test in  siriys xy (Autodesk Fusion 360 design; units mm, degrees)
Autodesk Fusion 360 part; units mm, degrees
note: some values were not read from the file. Set by a fixed rule: which sketch regions a step uses.
(part 1 of 2)
sketch "sdfjkvcsd" plane through (0, 0, 0) normal (0, 0, 1) x (1, 0, 0)
  line L0 (-177.8, 0) -> (0, 0)
  line L1 (-177.7996, 0.7937) -> (-177.8, 0)
  line L2 (0, 1.5875) -> (0.0008, 16.3703)
  line L3 (0.0008, 16.3703) -> (0, 48.914)
  line L4 (0, 48.914) -> (0, 81.4578)
  line L5 (0.0008, 101.1047) -> (0, 161.4297)
  line L6 (-177.8, 177.8) -> (-177.8, 1.5875)
  line L7 (0, 161.4297) -> (0.0008, 166.6875)
  line L8 (-177.8, 1.5875) -> (-177.7996, 0.7937)
  line L9 (0, 81.4578) -> (0.0008, 101.1047)
  line L10 (0, 0) -> (0, 1.5875)
  line L11 (0.0008, 166.6875) -> (0, 177.8)
  line L12 (0, 177.8) -> (-177.8, 177.8)
  line L13 (-157.7594, 165.1) -> (-134.3406, 165.1)
  line L14 (-134.3406, 114.3) -> (-157.7594, 114.3)
  line L15 (-157.7594, 114.3) -> (-157.7594, 165.1)
  line L16 (-134.3406, 165.1) -> (-134.3406, 114.3)
  line L17 (-76.0757, 98.8543) -> (-75.9232, 99.2225)
  line L18 (-25.4, 77.1906) -> (-73.6593, 77.1906)
  line L19 (-74.8124, 77.4674) -> (-75.153, 77.6757)
  line L20 (-75.7149, 99.5624) -> (-75.4561, 99.8654)
  line L21 (-74.4449, 77.3149) -> (-74.8124, 77.4674)
  line L22 (-74.0573, 77.2219) -> (-74.4449, 77.3149)
  line L23 (-75.7149, 78.2376) -> (-75.9232, 78.5775)
  line L24 (-75.9232, 99.2225) -> (-75.7149, 99.5624)
  line L25 (-75.153, 100.1243) -> (-74.8131, 100.3326)
  line L26 (-76.2, 79.7306) -> (-76.2, 98.0694)
  line L27 (-74.4449, 100.4851) -> (-74.0573, 100.5781)
  line L28 (-76.1687, 79.3333) -> (-76.2, 79.7306)
  line L29 (-75.153, 77.6757) -> (-75.4561, 77.9345)
  line L30 (-76.168, 98.4667) -> (-76.0757, 98.8543)
  line L31 (-75.4561, 99.8654) -> (-75.153, 100.1243)
  line L32 (-75.4561, 77.9345) -> (-75.7149, 78.2376)
  line L33 (-25.4, 100.6094) -> (-25.4, 77.1906)
  line L34 (-76.0757, 78.9457) -> (-76.1687, 79.3333)
  line L35 (-73.6593, 77.1906) -> (-74.0573, 77.2219)
  line L36 (-73.6593, 100.6094) -> (-25.4, 100.6094)
  line L37 (-74.8131, 100.3326) -> (-74.4449, 100.4851)
  line L38 (-74.0573, 100.5781) -> (-73.6593, 100.6094)
  line L39 (-75.9232, 78.5775) -> (-76.0757, 78.9457)
  line L40 (-76.2, 98.0694) -> (-76.168, 98.4667)
  line L41 (-75.7149, 75.153) -> (-75.4561, 75.456)
  line L42 (-75.1484, 75.7193) -> (-74.8086, 75.9276)
  line L43 (-76.1687, 74.0573) -> (-76.0757, 74.4449)
  line L44 (-26.0553, 73.1777) -> (-26.393, 72.9362)
  line L45 (-76.2, 73.6592) -> (-76.1687, 74.0573)
  line L46 (-76.2, 19.0544) -> (-76.2, 73.6592)
  line L47 (-75.3736, 75.5265) -> (-75.1484, 75.7193)
  line L48 (-75.9232, 74.8131) -> (-75.7149, 75.153)
  line L49 (-165.0955, 19.0544) -> (-76.2, 19.0544)
  line L50 (-74.0528, 76.1732) -> (-73.6555, 76.2037)
  line L51 (-165.0955, 19.05) -> (-165.0955, 19.0544)
  line L52 (-73.6555, 76.2037) -> (-25.3955, 76.2037)
  line L53 (-74.8086, 75.9276) -> (-74.4404, 76.0801)
  line L54 (-25.1866, 75.4706) -> (-25.1734, 75.4034)
  line L55 (-25.3355, 74.1805) -> (-25.4586, 73.9313)
  line L56 (-25.7615, 73.471) -> (-26.0553, 73.1777)
  line L57 (-25.5194, 73.809) -> (-25.7615, 73.471)
  line L58 (-75.4561, 75.456) -> (-75.3736, 75.5265)
  line L59 (-25.2531, 75.8137) -> (-25.2252, 75.6655)
  line L60 (-25.1602, 74.9892) -> (-25.2147, 74.5776)
  line L61 (-74.4404, 76.0801) -> (-74.0528, 76.1732)
  line L62 (-25.2147, 74.5776) -> (-25.3355, 74.1805)
  line L63 (-25.1734, 75.4034) -> (-25.1602, 74.9892)
  line L64 (-25.4586, 73.9313) -> (-25.5194, 73.809)
  line L65 (-25.3955, 76.2037) -> (-25.2531, 75.8137)
  line L66 (-76.0757, 74.4449) -> (-75.9232, 74.8131)
  line L67 (-25.2252, 75.6655) -> (-25.1866, 75.4706)
  line L68 (-46.9265, 66.04) -> (-46.9265, 12.7)
  line L69 (-31.6756, 73.2381) -> (-46.9265, 66.04)
  line L70 (-30.9503, 73.4556) -> (-31.3211, 73.374)
  line L71 (-31.3211, 73.374) -> (-31.6756, 73.2381)
  line L72 (-165.1, 16.3703) -> (-165.0993, 19.05)
  line L73 (-165.1, 12.7) -> (-165.1, 16.3703)
  line L74 (-29.8238, 73.3623) -> (-30.1932, 73.4497)
  line L75 (-30.5716, 73.481) -> (-30.9503, 73.4556)
  line L76 (-27.1628, 72.6327) -> (-27.5744, 72.5788)
  line L77 (-27.9893, 72.5927) -> (-28.3964, 72.6741)
  line L78 (-26.393, 72.9362) -> (-26.7654, 72.7529)
  line L79 (-26.7654, 72.7529) -> (-27.1628, 72.6327)
  line L80 (-27.5744, 72.5788) -> (-27.9893, 72.5927)
  line L81 (-30.1932, 73.4497) -> (-30.5716, 73.481)
  line L82 (-28.6779, 72.7803) -> (-28.7841, 72.8206)
  line L83 (-165.0993, 19.05) -> (-165.0955, 19.05)
  line L84 (-46.9265, 12.7) -> (-165.1, 12.7)
  line L85 (-28.3964, 72.6741) -> (-28.6779, 72.7803)
  line L86 (-28.7841, 72.8206) -> (-29.1442, 73.0285)
  line L87 (-29.4715, 73.2209) -> (-29.8238, 73.3623)
  line L88 (-29.1442, 73.0285) -> (-29.4715, 73.2209)
  line L89 (-74.0545, 152.3825) -> (-73.8095, 152.2578)
  line L90 (-72.599, 150.1924) -> (-72.6167, 149.7776)
  line L91 (-75.1522, 102.0851) -> (-75.4553, 102.344)
  line L92 (-75.4553, 102.344) -> (-75.7149, 102.647)
  line L93 (-19.05, 12.7) -> (-19.05, 101.6)
  line L94 (-75.8093, 152.5423) -> (-75.4013, 152.6192)
  line L95 (-73.296, 146.0975) -> (-66.04, 130.3494)
  line L96 (-16.3703, 130.3501) -> (-12.7, 130.3501)
  line L97 (-72.649, 150.6045) -> (-72.599, 150.1924)
  line L98 (-74.9869, 152.6287) -> (-74.576, 152.5704)
  line L99 (-73.5287, 147.2036) -> (-73.5068, 146.8247)
  line L100 (-73.0631, 148.6268) -> (-73.2584, 148.3013)
  line L101 (-76.1993, 152.4) -> (-75.8093, 152.5423)
  line L102 (-66.04, 130.3494) -> (-16.3703, 130.3501)
  line L103 (-75.4013, 152.6192) -> (-74.9869, 152.6287)
  line L104 (-12.7, 130.3501) -> (-12.7, 12.7)
  line L105 (-73.1839, 151.7169) -> (-73.0434, 151.5167)
  line L106 (-16.371, 12.7) -> (-19.05, 12.7)
  line L107 (-73.0434, 151.5167) -> (-72.9455, 151.3763)
  line L108 (-72.8519, 148.9842) -> (-73.0631, 148.6268)
  line L109 (-74.576, 152.5704) -> (-74.18, 152.4459)
  line L110 (-73.4031, 147.9503) -> (-73.4939, 147.5817)
  line L111 (-73.6593, 101.6) -> (-74.0573, 101.6313)
  line L112 (-76.0757, 103.3551) -> (-76.1687, 103.7427)
  line L113 (-73.2584, 148.3013) -> (-73.4031, 147.9503)
  line L114 (-73.4939, 147.5817) -> (-73.5287, 147.2036)
  line L115 (-72.9455, 151.3763) -> (-72.7656, 151.0029)
  line L116 (-72.7018, 149.3713) -> (-72.8519, 148.9842)
  line L117 (-73.5068, 146.8247) -> (-73.4286, 146.4532)
  line L118 (-73.8095, 152.2578) -> (-73.4745, 152.0134)
  line L119 (-75.7149, 102.647) -> (-75.9232, 102.9869)
  line L120 (-75.9232, 102.9869) -> (-76.0757, 103.3551)
  line L121 (-19.05, 101.6) -> (-73.6593, 101.6)
  line L122 (-16.3703, 12.7) -> (-16.371, 12.7)
  line L123 (-72.6167, 149.7776) -> (-72.7018, 149.3713)
  line L124 (-73.4286, 146.4532) -> (-73.296, 146.0975)
  line L125 (-74.0573, 101.6313) -> (-74.4449, 101.7243)
  line L126 (-76.1687, 103.7427) -> (-76.1993, 104.14)
  line L127 (-76.1993, 104.14) -> (-76.1993, 152.4)
  line L128 (-72.7656, 151.0029) -> (-72.649, 150.6045)
  line L129 (-74.18, 152.4459) -> (-74.0545, 152.3825)
  line L130 (-74.4449, 101.7243) -> (-74.8124, 101.8768)
  line L131 (-74.8124, 101.8768) -> (-75.1522, 102.0851)
  line L132 (-12.7, 12.7) -> (-16.3703, 12.7)
  line L133 (-73.4745, 152.0134) -> (-73.1839, 151.7169)
  line L134 (-45.9359, 16.3703) -> (-45.9359, 63.5)
  line L135 (-45.9359, 63.5) -> (-20.0406, 63.5)
  line L136 (-20.0406, 63.5) -> (-20.0406, 12.7)
  line L137 (-20.0406, 12.7) -> (-45.9352, 12.7)
  line L138 (-45.9352, 12.7) -> (-45.9359, 16.3703)
  line L139 (-80.1666, 90.9976) -> (-79.8464, 90.5647)
  line L140 (-84.5446, 91.3703) -> (-84.0984, 91.6711)
  line L141 (-84.9334, 90.9976) -> (-84.5446, 91.3703)
  line L142 (-80.5554, 91.3703) -> (-80.1666, 90.9976)
  line L143 (-83.6077, 91.8936) -> (-83.0866, 92.0293)
  line L144 (-81.4923, 91.8936) -> (-81.0016, 91.6718)
  line L145 (-79.3779, 89.0348) -> (-79.4007, 88.4967)
  line L146 (-82.0134, 92.0293) -> (-81.4923, 91.8936)
  line L147 (-81.2422, 86.0069) -> (-81.75, 85.8274)
  line L148 (-81.75, 85.8274) -> (-82.2807, 85.7364)
  line L149 (-79.715, 87.4706) -> (-79.9973, 87.012)
  line L150 (-85.5858, 87.9703) -> (-85.6993, 88.4967)
  line L151 (-84.7469, 86.6078) -> (-85.1027, 87.012)
  line L152 (-85.1027, 87.012) -> (-85.385, 87.4706)
  line L153 (-85.385, 87.4706) -> (-85.5858, 87.9703)
  line L154 (-85.6537, 89.5689) -> (-85.4961, 90.0838)
  line L155 (-79.9973, 87.012) -> (-80.3531, 86.6078)
  line L156 (-79.5142, 87.9703) -> (-79.715, 87.4706)
  line L157 (-79.604, 90.0838) -> (-79.4463, 89.5689)
  line L158 (-82.55, 92.075) -> (-82.0134, 92.0293)
  line L159 (-81.0016, 91.6718) -> (-80.5554, 91.3703)
  line L160 (-85.6993, 88.4967) -> (-85.7221, 89.0348)
  line L161 (-83.3493, 85.8274) -> (-83.857, 86.0069)
  line L162 (-83.0866, 92.0293) -> (-82.55, 92.075)
  line L163 (-82.8193, 85.7364) -> (-83.3493, 85.8274)
  line L164 (-85.2536, 90.5647) -> (-84.9334, 90.9976)
  line L165 (-84.3279, 86.2695) -> (-84.7469, 86.6078)
  line L166 (-83.857, 86.0069) -> (-84.3279, 86.2695)
  line L167 (-80.7721, 86.2695) -> (-81.2422, 86.0069)
  line L168 (-85.4961, 90.0838) -> (-85.2536, 90.5647)
  line L169 (-82.2807, 85.7364) -> (-82.8193, 85.7364)
  line L170 (-85.7221, 89.0348) -> (-85.6537, 89.5689)
  line L171 (-79.4007, 88.4967) -> (-79.5142, 87.9703)
  line L172 (-84.0984, 91.6711) -> (-83.6077, 91.8936)
  line L173 (-80.3531, 86.6078) -> (-80.7721, 86.2695)
  line L174 (-79.8464, 90.5647) -> (-79.604, 90.0838)
  line L175 (-79.4463, 89.5689) -> (-79.3779, 89.0348)
  line L176 (-168.3007, 5.9467) -> (-168.4142, 5.4203)
  line L177 (-174.5537, 7.0189) -> (-174.396, 7.5338)
  line L178 (-168.7464, 8.0147) -> (-168.504, 7.5338)
  line L179 (-171.7193, 3.1864) -> (-172.25, 3.2774)
  line L180 (-174.396, 7.5338) -> (-174.1536, 8.0147)
  line L181 (-170.1422, 3.4568) -> (-170.65, 3.2774)
  line L182 (-172.7578, 3.4568) -> (-173.2279, 3.7195)
  line L183 (-174.1536, 8.0147) -> (-173.8334, 8.4476)
  line L184 (-174.2843, 4.9206) -> (-174.4858, 5.4203)
  line L185 (-171.1807, 3.1864) -> (-171.7193, 3.1864)
  line L186 (-174.0027, 4.462) -> (-174.2843, 4.9206)
  line L187 (-172.25, 3.2774) -> (-172.7578, 3.4568)
  line L188 (-168.504, 7.5338) -> (-168.3463, 7.0189)
  line L189 (-171.45, 9.525) -> (-170.9134, 9.4793)
  line L190 (-171.9866, 9.4793) -> (-171.45, 9.525)
  line L191 (-168.615, 4.9206) -> (-168.8973, 4.462)
  line L192 (-174.5993, 5.9467) -> (-174.6222, 6.4847)
  line L193 (-173.8334, 8.4476) -> (-173.4446, 8.8203)
  line L194 (-172.9984, 9.1218) -> (-172.5077, 9.3436)
  line L195 (-168.3463, 7.0189) -> (-168.2779, 6.4847)
  line L196 (-169.2531, 4.0578) -> (-169.6721, 3.7195)
  line L197 (-173.2279, 3.7195) -> (-173.6469, 4.0578)
  line L198 (-169.6721, 3.7195) -> (-170.1422, 3.4568)
  line L199 (-169.9016, 9.1218) -> (-169.4554, 8.8203)
  line L200 (-174.4858, 5.4203) -> (-174.5993, 5.9467)
  line L201 (-169.0666, 8.4476) -> (-168.7464, 8.0147)
  line L202 (-173.6469, 4.0578) -> (-174.0027, 4.462)
  line L203 (-170.3923, 9.3436) -> (-169.9016, 9.1218)
  line L204 (-170.9134, 9.4793) -> (-170.3923, 9.3436)
  line L205 (-173.4446, 8.8203) -> (-172.9984, 9.1218)
  line L206 (-174.6222, 6.4847) -> (-174.5537, 7.0189)
  line L207 (-168.2779, 6.4847) -> (-168.3007, 5.9467)
  line L208 (-172.5077, 9.3436) -> (-171.9866, 9.4793)
  line L209 (-170.65, 3.2774) -> (-171.1807, 3.1864)
  line L210 (-168.4142, 5.4203) -> (-168.615, 4.9206)
  line L211 (-168.8973, 4.462) -> (-169.2531, 4.0578)
  line L212 (-169.4554, 8.8203) -> (-169.0666, 8.4476)
  line L213 (-97.2446, 91.3703) -> (-96.7984, 91.6718)
  line L214 (-93.9422, 86.0069) -> (-94.45, 85.8274)
  line L215 (-93.2554, 91.3703) -> (-92.8666, 90.9976)
  line L216 (-97.0272, 86.2695) -> (-97.4462, 86.6078)
  line L217 (-97.6334, 90.9976) -> (-97.2446, 91.3703)
  line L218 (-98.085, 87.4706) -> (-98.2858, 87.9703)
  line L219 (-92.8666, 90.9976) -> (-92.5464, 90.5647)
  line L220 (-98.3993, 88.4967) -> (-98.4214, 89.0348)
  line L221 (-94.45, 85.8274) -> (-94.9807, 85.7364)
  line L222 (-96.05, 85.8274) -> (-96.5578, 86.0069)
  line L223 (-92.2142, 87.9703) -> (-92.415, 87.4706)
  line L224 (-95.25, 92.075) -> (-94.7134, 92.0293)
  line L225 (-92.5464, 90.5647) -> (-92.304, 90.0838)
  line L226 (-96.5578, 86.0069) -> (-97.0272, 86.2695)
  line L227 (-92.1007, 88.4967) -> (-92.2142, 87.9703)
  line L228 (-94.9807, 85.7364) -> (-95.5193, 85.7364)
  line L229 (-92.6973, 87.012) -> (-93.0531, 86.6078)
  line L230 (-93.7016, 91.6718) -> (-93.2554, 91.3703)
  line L231 (-94.1923, 91.8936) -> (-93.7016, 91.6718)
  line L232 (-98.4214, 89.0348) -> (-98.353, 89.5689)
  line L233 (-97.8027, 87.012) -> (-98.085, 87.4706)
  line L234 (-94.7134, 92.0293) -> (-94.1923, 91.8936)
  line L235 (-98.2858, 87.9703) -> (-98.3993, 88.4967)
  line L236 (-92.415, 87.4706) -> (-92.6973, 87.012)
  line L237 (-95.5193, 85.7364) -> (-96.05, 85.8274)
  line L238 (-92.0779, 89.0348) -> (-92.1007, 88.4967)
  line L239 (-93.4721, 86.2695) -> (-93.9422, 86.0069)
  line L240 (-92.1463, 89.5689) -> (-92.0779, 89.0348)
  line L241 (-98.353, 89.5689) -> (-98.196, 90.0838)
  line L242 (-97.9536, 90.5647) -> (-97.6334, 90.9976)
  line L243 (-95.7866, 92.0293) -> (-95.25, 92.075)
  line L244 (-97.4462, 86.6078) -> (-97.8027, 87.012)
  line L245 (-96.3077, 91.8936) -> (-95.7866, 92.0293)
  line L246 (-96.7984, 91.6718) -> (-96.3077, 91.8936)
  line L247 (-98.196, 90.0838) -> (-97.9536, 90.5647)
  line L248 (-93.0531, 86.6078) -> (-93.4721, 86.2695)
  line L249 (-92.304, 90.0838) -> (-92.1463, 89.5689)
  line L250 (-100.6094, 104.14) -> (-100.6094, 152.3992)
  line L251 (-99.2225, 101.8768) -> (-99.5624, 102.0851)
  line L252 (-79.3333, 101.6313) -> (-79.7306, 101.6)
  line L253 (-78.2828, 152.4) -> (-77.1906, 152.4)
  line L254 (-77.2219, 103.7427) -> (-77.3149, 103.3551)
  line L255 (-98.0694, 101.6) -> (-98.4667, 101.6313)
  line L256 (-79.7306, 101.6) -> (-98.0694, 101.6)
  line L257 (-100.1243, 102.647) -> (-100.3318, 102.9869)
  line L258 (-100.3318, 102.9869) -> (-100.4851, 103.3551)
  line L259 (-77.3149, 103.3551) -> (-77.4674, 102.9869)
  line L260 (-100.5781, 103.7427) -> (-100.6094, 104.14)
  line L261 (-99.5624, 102.0851) -> (-99.8654, 102.344)
  line L262 (-77.1906, 104.14) -> (-77.2219, 103.7427)
  line L263 (-77.6757, 102.647) -> (-77.9345, 102.344)
  line L264 (-78.5775, 101.8768) -> (-78.9457, 101.7243)
  line L265 (-77.1906, 152.4) -> (-77.1906, 104.14)
  line L266 (-78.9457, 101.7243) -> (-79.3333, 101.6313)
  line L267 (-77.4674, 102.9869) -> (-77.6757, 102.647)
  line L268 (-77.9345, 102.344) -> (-78.2376, 102.0851)
  line L269 (-100.4851, 103.3551) -> (-100.5781, 103.7427)
  line L270 (-99.8654, 102.344) -> (-100.1243, 102.647)
  line L271 (-98.4667, 101.6313) -> (-98.8543, 101.7243)
  line L272 (-98.8543, 101.7243) -> (-99.2225, 101.8768)
  line L273 (-100.6094, 152.3992) -> (-78.2828, 152.4)
  line L274 (-78.2376, 102.0851) -> (-78.5775, 101.8768)
  line L275 (-12.7, 157.7594) -> (-12.6996, 144.5501)
  line L276 (-63.5, 157.7594) -> (-12.7, 157.7594)
  line L277 (-63.5, 131.3407) -> (-63.5, 157.7594)
  line L278 (-12.6996, 144.5501) -> (-12.7, 131.3407)
  line L279 (-12.7, 131.3407) -> (-63.5, 131.3407)
  line L280 (-77.1906, 25.4) -> (-100.6094, 25.4)
  line L281 (-77.4674, 74.8131) -> (-77.3149, 74.4449)
  line L282 (-77.1906, 73.66) -> (-77.1906, 25.4)
  line L283 (-79.3333, 76.1687) -> (-78.9457, 76.0757)
  line L284 (-99.2225, 75.9232) -> (-98.8543, 76.0757)
  line L285 (-79.7306, 76.2) -> (-79.3333, 76.1687)
  line L286 (-78.5775, 75.9232) -> (-78.2376, 75.7149)
  line L287 (-78.2376, 75.7149) -> (-77.9345, 75.456)
  line L288 (-78.9457, 76.0757) -> (-78.5775, 75.9232)
  line L289 (-77.6757, 75.153) -> (-77.4674, 74.8131)
  line L290 (-100.6094, 25.4) -> (-100.6094, 73.6592)
  line L291 (-77.3149, 74.4449) -> (-77.2219, 74.0573)
  line L292 (-100.5781, 74.0573) -> (-100.4851, 74.4449)
  line L293 (-77.9345, 75.456) -> (-77.6757, 75.153)
  line L294 (-77.2219, 74.0573) -> (-77.1906, 73.66)
  line L295 (-98.8543, 76.0757) -> (-98.4667, 76.1687)
  line L296 (-100.3326, 74.8131) -> (-100.1243, 75.153)
  line L297 (-100.1243, 75.153) -> (-99.8654, 75.4553)
  line L298 (-98.4667, 76.1687) -> (-98.0694, 76.2)
  line L299 (-99.5624, 75.7149) -> (-99.2225, 75.9232)
  line L300 (-99.8654, 75.4553) -> (-99.5624, 75.7149)
  line L301 (-98.0694, 76.2) -> (-79.7306, 76.2)
  line L302 (-100.6094, 73.6592) -> (-100.5781, 74.0573)
  line L303 (-100.4851, 74.4449) -> (-100.3326, 74.8131)
  line L304 (-102.9869, 100.3326) -> (-102.647, 100.1243)
  line L305 (-101.6, 79.7306) -> (-101.6313, 79.3333)
  line L306 (-104.14, 100.6094) -> (-103.7427, 100.5781)
  line L307 (-102.647, 100.1243) -> (-102.344, 99.8654)
  line L308 (-101.8769, 99.2225) -> (-101.7243, 98.8543)
  line L309 (-152.4, 100.6094) -> (-104.14, 100.6094)
  line L310 (-102.0851, 78.2376) -> (-102.344, 77.9345)
  line L311 (-103.7427, 100.5781) -> (-103.3551, 100.4851)
  line L312 (-102.344, 99.8654) -> (-102.0851, 99.5624)
  line L313 (-103.3551, 100.4851) -> (-102.9869, 100.3326)
  line L314 (-152.4, 81.4578) -> (-152.4, 100.6094)
  line L315 (-102.0851, 99.5624) -> (-101.8769, 99.2225)
  line L316 (-102.647, 77.6757) -> (-102.9869, 77.4674)
  line L317 (-101.7243, 78.9457) -> (-101.8769, 78.5775)
  line L318 (-101.6313, 79.3333) -> (-101.7243, 78.9457)
  line L319 (-101.8769, 78.5775) -> (-102.0851, 78.2376)
  line L320 (-101.7243, 98.8543) -> (-101.6313, 98.4667)
  line L321 (-103.3551, 77.3149) -> (-103.7427, 77.2219)
  line L322 (-101.6313, 98.4667) -> (-101.6, 98.0694)
  line L323 (-102.9869, 77.4674) -> (-103.3551, 77.3149)
  line L324 (-152.3993, 77.1906) -> (-152.4, 81.4578)
  line L325 (-101.6, 98.0694) -> (-101.6, 79.7306)
  line L326 (-103.7427, 77.2219) -> (-104.14, 77.1906)
  line L327 (-102.344, 77.9345) -> (-102.647, 77.6757)
  line L328 (-104.14, 77.1906) -> (-152.3993, 77.1906)
  line L329 (-114.3, 20.0406) -> (-165.1, 20.0406)
  line L330 (-165.1, 43.4594) -> (-114.3, 43.4594)
  line L331 (-165.1, 20.0406) -> (-165.1, 43.4594)
  line L332 (-114.3, 43.4594) -> (-114.3, 20.0406)
  line L333 (-4.3554, 8.8203) -> (-3.9666, 8.4476)
  line L334 (-8.9019, 4.462) -> (-9.185, 4.9206)
  line L335 (-9.0536, 8.0147) -> (-8.7334, 8.4476)
  line L336 (-4.1531, 4.0578) -> (-4.5721, 3.7195)
  line L337 (-8.1279, 3.7195) -> (-8.5469, 4.0578)
  line L338 (-5.55, 3.2774) -> (-6.0807, 3.1864)
  line L339 (-9.2961, 7.5338) -> (-9.0536, 8.0147)
  line L340 (-6.0807, 3.1864) -> (-6.6193, 3.1864)
  line L341 (-7.657, 3.4568) -> (-8.1279, 3.7195)
  line L342 (-3.7973, 4.462) -> (-4.1531, 4.0578)
  line L343 (-9.5221, 6.4847) -> (-9.4537, 7.0189)
  line L344 (-5.8134, 9.4793) -> (-5.2923, 9.3436)
  line L345 (-3.1779, 6.4847) -> (-3.2007, 5.9467)
  line L346 (-3.6464, 8.0147) -> (-3.404, 7.5338)
  line L347 (-3.2463, 7.0189) -> (-3.1779, 6.4847)
  line L348 (-7.15, 3.2774) -> (-7.657, 3.4568)
  line L349 (-9.4537, 7.0189) -> (-9.2961, 7.5338)
  line L350 (-4.5721, 3.7195) -> (-5.0422, 3.4568)
  line L351 (-7.4077, 9.3436) -> (-6.8866, 9.4793)
  line L352 (-3.2007, 5.9467) -> (-3.3142, 5.4203)
  line L353 (-9.3858, 5.4203) -> (-9.4993, 5.9467)
  line L354 (-8.5469, 4.0578) -> (-8.9019, 4.462)
  line L355 (-3.404, 7.5338) -> (-3.2463, 7.0189)
  line L356 (-8.7334, 8.4476) -> (-8.3446, 8.8203)
  line L357 (-7.8984, 9.1218) -> (-7.4077, 9.3436)
  line L358 (-6.8866, 9.4793) -> (-6.35, 9.525)
  line L359 (-9.185, 4.9206) -> (-9.3858, 5.4203)
  line L360 (-5.2923, 9.3436) -> (-4.8016, 9.1218)
  line L361 (-3.9666, 8.4476) -> (-3.6464, 8.0147)
  line L362 (-8.3446, 8.8203) -> (-7.8984, 9.1218)
  line L363 (-9.4993, 5.9467) -> (-9.5221, 6.4847)
  line L364 (-4.8016, 9.1218) -> (-4.3554, 8.8203)
  line L365 (-3.515, 4.9206) -> (-3.7973, 4.462)
  line L366 (-3.3142, 5.4203) -> (-3.515, 4.9206)
  line L367 (-6.35, 9.525) -> (-5.8134, 9.4793)
  line L368 (-5.0422, 3.4568) -> (-5.55, 3.2774)
  line L369 (-6.6193, 3.1864) -> (-7.15, 3.2774)
  line L370 (-172.7578, 168.5569) -> (-173.2279, 168.8195)
  line L371 (-174.4858, 170.5203) -> (-174.5993, 171.0467)
  line L372 (-172.25, 168.3774) -> (-172.7578, 168.5569)
  line L373 (-172.9984, 174.2211) -> (-172.5077, 174.4436)
  line L374 (-171.9866, 174.5793) -> (-171.45, 174.625)
  line L375 (-173.8334, 173.5476) -> (-173.4446, 173.9203)
  line L376 (-169.9016, 174.2218) -> (-169.4554, 173.9203)
  line L377 (-174.285, 170.0206) -> (-174.4858, 170.5203)
  line L378 (-169.6721, 168.8195) -> (-170.1422, 168.5569)
  line L379 (-173.6469, 169.1578) -> (-174.0027, 169.5621)
  line L380 (-170.65, 168.3774) -> (-171.1807, 168.2864)
  line L381 (-171.45, 174.625) -> (-170.9134, 174.5793)
  line L382 (-174.1536, 173.1147) -> (-173.8334, 173.5476)
  line L383 (-174.5993, 171.0467) -> (-174.6222, 171.5848)
  line L384 (-173.4446, 173.9203) -> (-172.9984, 174.2211)
  line L385 (-172.5077, 174.4436) -> (-171.9866, 174.5793)
  line L386 (-174.6222, 171.5848) -> (-174.5537, 172.1189)
  line L387 (-171.1807, 168.2864) -> (-171.7193, 168.2864)
  line L388 (-168.2779, 171.5848) -> (-168.3007, 171.0467)
  line L389 (-168.615, 170.0206) -> (-168.8973, 169.5621)
  line L390 (-173.2279, 168.8195) -> (-173.6469, 169.1578)
  line L391 (-168.3007, 171.0467) -> (-168.4142, 170.5203)
  line L392 (-168.4142, 170.5203) -> (-168.615, 170.0206)
  line L393 (-168.504, 172.6338) -> (-168.3463, 172.1189)
  line L394 (-171.7193, 168.2864) -> (-172.25, 168.3774)
  line L395 (-170.9134, 174.5793) -> (-170.3923, 174.4436)
  line L396 (-169.4554, 173.9203) -> (-169.0666, 173.5476)
  line L397 (-170.3923, 174.4436) -> (-169.9016, 174.2218)
  line L398 (-168.8973, 169.5621) -> (-169.2531, 169.1578)
  line L399 (-174.396, 172.6338) -> (-174.1536, 173.1147)
  line L400 (-170.1422, 168.5569) -> (-170.65, 168.3774)
  line L401 (-174.5537, 172.1189) -> (-174.396, 172.6338)
  line L402 (-174.0027, 169.5621) -> (-174.285, 170.0206)
  line L403 (-168.7464, 173.1147) -> (-168.504, 172.6338)
  line L404 (-169.0666, 173.5476) -> (-168.7464, 173.1147)
  line L405 (-169.2531, 169.1578) -> (-169.6721, 168.8195)
  line L406 (-168.3463, 172.1189) -> (-168.2779, 171.5848)
  line L407 (-145.7807, 168.2864) -> (-146.3193, 168.2864)
  line L408 (-145.5134, 174.5793) -> (-144.9923, 174.4436)
  line L409 (-148.6027, 169.5621) -> (-148.885, 170.0206)
  line L410 (-148.2469, 169.1578) -> (-148.6027, 169.5621)
  line L411 (-149.1537, 172.1189) -> (-148.996, 172.6338)
  line L412 (-148.885, 170.0206) -> (-149.0851, 170.5203)
  line L413 (-143.215, 170.0206) -> (-143.4973, 169.5621)
  line L414 (-142.9463, 172.1189) -> (-142.8779, 171.5848)
  line L415 (-144.9923, 174.4436) -> (-144.5016, 174.2218)
  line L416 (-142.9007, 171.0467) -> (-143.0142, 170.5203)
  line L417 (-149.0851, 170.5203) -> (-149.1993, 171.0467)
  line L418 (-144.5016, 174.2218) -> (-144.0554, 173.9203)
  line L419 (-148.996, 172.6338) -> (-148.7536, 173.1147)
  line L420 (-144.2721, 168.8195) -> (-144.7422, 168.5569)
  line L421 (-143.4973, 169.5621) -> (-143.8531, 169.1578)
  line L422 (-146.0496, 174.625) -> (-145.5134, 174.5793)
  line L423 (-146.5866, 174.5793) -> (-146.0496, 174.625)
  line L424 (-147.8279, 168.8195) -> (-148.2469, 169.1578)
  line L425 (-149.2221, 171.5848) -> (-149.1537, 172.1189)
  line L426 (-144.7422, 168.5569) -> (-145.25, 168.3774)
  line L427 (-143.3464, 173.1147) -> (-143.1039, 172.6338)
  line L428 (-142.8779, 171.5848) -> (-142.9007, 171.0467)
  line L429 (-143.6666, 173.5476) -> (-143.3464, 173.1147)
  line L430 (-148.0446, 173.9203) -> (-147.5984, 174.2218)
  line L431 (-143.1039, 172.6338) -> (-142.9463, 172.1189)
  line L432 (-146.3193, 168.2864) -> (-146.85, 168.3774)
  line L433 (-144.0554, 173.9203) -> (-143.6666, 173.5476)
  line L434 (-143.0142, 170.5203) -> (-143.215, 170.0206)
  line L435 (-146.85, 168.3774) -> (-147.3578, 168.5569)
  line L436 (-149.1993, 171.0467) -> (-149.2221, 171.5848)
  line L437 (-148.4334, 173.5476) -> (-148.0446, 173.9203)
  line L438 (-143.8531, 169.1578) -> (-144.2721, 168.8195)
  line L439 (-147.3578, 168.5569) -> (-147.8279, 168.8195)
  line L440 (-148.7536, 173.1147) -> (-148.4334, 173.5476)
  line L441 (-147.5984, 174.2218) -> (-147.1077, 174.4436)
  line L442 (-145.25, 168.3774) -> (-145.7807, 168.2864)
  line L443 (-147.1077, 174.4436) -> (-146.5866, 174.5793)
  line L444 (-91.735, 4.9206) -> (-91.9358, 5.4203)
  line L445 (-88.3634, 9.4793) -> (-87.8423, 9.3436)
  line L446 (-87.1221, 3.7195) -> (-87.5922, 3.4568)
  line L447 (-89.1693, 3.1864) -> (-89.7, 3.2774)
  line L448 (-86.065, 4.9206) -> (-86.3473, 4.462)
  line L449 (-88.9, 9.525) -> (-88.3634, 9.4793)
  line L450 (-92.0037, 7.0189) -> (-91.846, 7.5338)
  line L451 (-87.5922, 3.4568) -> (-88.1, 3.2774)
  line L452 (-91.2834, 8.4476) -> (-90.8946, 8.8203)
  line L453 (-92.0721, 6.4847) -> (-92.0037, 7.0189)
  line L454 (-86.1964, 8.0147) -> (-85.954, 7.5338)
  line L455 (-85.7963, 7.0189) -> (-85.7279, 6.4847)
  line L456 (-86.9054, 8.8203) -> (-86.5166, 8.4476)
  line L457 (-87.8423, 9.3436) -> (-87.3516, 9.1218)
  line L458 (-89.7, 3.2774) -> (-90.207, 3.4568)
  line L459 (-90.6779, 3.7195) -> (-91.0969, 4.0578)
  line L460 (-86.5166, 8.4476) -> (-86.1964, 8.0147)
  line L461 (-88.1, 3.2774) -> (-88.6307, 3.1864)
  line L462 (-91.846, 7.5338) -> (-91.6036, 8.0147)
  line L463 (-91.0969, 4.0578) -> (-91.4527, 4.462)
  line L464 (-91.6036, 8.0147) -> (-91.2834, 8.4476)
  line L465 (-89.9577, 9.3436) -> (-89.4366, 9.4793)
  line L466 (-85.954, 7.5338) -> (-85.7963, 7.0189)
  line L467 (-89.4366, 9.4793) -> (-88.9, 9.525)
  line L468 (-90.4484, 9.1218) -> (-89.9577, 9.3436)
  line L469 (-86.3473, 4.462) -> (-86.7031, 4.0578)
  line L470 (-85.8642, 5.4203) -> (-86.065, 4.9206)
  line L471 (-90.8946, 8.8203) -> (-90.4484, 9.1218)
  line L472 (-91.4527, 4.462) -> (-91.735, 4.9206)
  line L473 (-90.207, 3.4568) -> (-90.6779, 3.7195)
  line L474 (-86.7031, 4.0578) -> (-87.1221, 3.7195)
  line L475 (-92.0493, 5.9467) -> (-92.0721, 6.4847)
  line L476 (-88.6307, 3.1864) -> (-89.1693, 3.1864)
  line L477 (-87.3516, 9.1218) -> (-86.9054, 8.8203)
  line L478 (-85.7279, 6.4847) -> (-85.7507, 5.9467)
  line L479 (-91.9358, 5.4203) -> (-92.0493, 5.9467)
  line L480 (-85.7507, 5.9467) -> (-85.8642, 5.4203)
  line L481 (-9.0536, 173.1147) -> (-8.7334, 173.5476)
  line L482 (-6.8866, 174.5793) -> (-6.35, 174.625)
  line L483 (-3.6464, 173.1147) -> (-3.404, 172.6338)
  line L484 (-5.8134, 174.5793) -> (-5.2923, 174.4436)
  line L485 (-4.8016, 174.2218) -> (-4.3554, 173.9203)
  line L486 (-4.5721, 168.8195) -> (-5.0422, 168.5569)
  line L487 (-4.1531, 169.1578) -> (-4.5721, 168.8195)
  line L488 (-3.404, 172.6338) -> (-3.2463, 172.1181)
  line L489 (-5.0422, 168.5569) -> (-5.55, 168.3774)
  line L490 (-3.3142, 170.5203) -> (-3.515, 170.0206)
  line L491 (-3.9666, 173.5476) -> (-3.6464, 173.1147)
  line L492 (-3.2463, 172.1181) -> (-3.1779, 171.5848)
  line L493 (-6.35, 174.625) -> (-5.8134, 174.5793)
  line L494 (-5.2923, 174.4436) -> (-4.8016, 174.2218)
  line L495 (-3.1779, 171.5848) -> (-3.2007, 171.0467)
  line L496 (-7.4077, 174.4436) -> (-6.8866, 174.5793)
  line L497 (-4.3554, 173.9203) -> (-3.9666, 173.5476)
  line L498 (-3.7973, 169.5621) -> (-4.1531, 169.1578)
  line L499 (-3.515, 170.0206) -> (-3.7973, 169.5621)
  line L500 (-5.55, 168.3774) -> (-6.0807, 168.2864)
  line L501 (-6.0807, 168.2864) -> (-6.6193, 168.2864)
  line L502 (-6.6193, 168.2864) -> (-7.15, 168.3774)
  line L503 (-9.5221, 171.5848) -> (-9.4537, 172.1189)
  line L504 (-8.3446, 173.9203) -> (-7.8984, 174.2218)
  line L505 (-7.8984, 174.2218) -> (-7.4077, 174.4436)
  line L506 (-9.2961, 172.6338) -> (-9.0536, 173.1147)
  line L507 (-8.1279, 168.8195) -> (-8.5469, 169.1578)
  line L508 (-9.185, 170.0206) -> (-9.3858, 170.5203)
  line L509 (-9.3858, 170.5203) -> (-9.4993, 171.0467)
  line L510 (-8.5469, 169.1578) -> (-8.9027, 169.5621)
  line L511 (-7.15, 168.3774) -> (-7.6578, 168.5569)
  line L512 (-7.6578, 168.5569) -> (-8.1279, 168.8195)
  line L513 (-8.9027, 169.5621) -> (-9.185, 170.0206)
  line L514 (-9.4537, 172.1189) -> (-9.2961, 172.6338)
  line L515 (-3.2007, 171.0467) -> (-3.3142, 170.5203)
  line L516 (-8.7334, 173.5476) -> (-8.3446, 173.9203)
  line L517 (-9.4993, 171.0467) -> (-9.5221, 171.5848)
  line L518 (-143.3464, 8.0147) -> (-143.1039, 7.5338)
  line L519 (-143.1039, 7.5338) -> (-142.9463, 7.0189)
  line L520 (-148.4334, 8.4476) -> (-148.0446, 8.8203)
  line L521 (-142.9463, 7.0189) -> (-142.8779, 6.4847)
  line L522 (-143.6666, 8.4476) -> (-143.3464, 8.0147)
  line L523 (-143.8531, 4.0578) -> (-144.2721, 3.7195)
  line L524 (-144.9923, 9.3429) -> (-144.5016, 9.1218)
  line L525 (-146.05, 9.525) -> (-145.5134, 9.4793)
  line L526 (-145.5134, 9.4793) -> (-144.9923, 9.3429)
  line L527 (-144.5016, 9.1218) -> (-144.0554, 8.8203)
  line L528 (-142.8779, 6.4847) -> (-142.9007, 5.9467)
  line L529 (-143.215, 4.9206) -> (-143.4973, 4.462)
  line L530 (-147.1077, 9.3436) -> (-146.5866, 9.4793)
  line L531 (-143.4973, 4.462) -> (-143.8531, 4.0578)
  line L532 (-149.1537, 7.0189) -> (-148.996, 7.5338)
  line L533 (-144.2721, 3.7195) -> (-144.7422, 3.4568)
  line L534 (-144.7422, 3.4568) -> (-145.25, 3.2774)
  line L535 (-144.0554, 8.8203) -> (-143.6666, 8.4476)
  line L536 (-145.7807, 3.1864) -> (-146.3193, 3.1864)
  line L537 (-147.5984, 9.1218) -> (-147.1077, 9.3436)
  line L538 (-142.9007, 5.9467) -> (-143.0142, 5.4203)
  line L539 (-146.5866, 9.4793) -> (-146.05, 9.525)
  line L540 (-143.0142, 5.4203) -> (-143.215, 4.9206)
  line L541 (-145.25, 3.2774) -> (-145.7807, 3.1864)
  line L542 (-148.0446, 8.8203) -> (-147.5984, 9.1218)
  line L543 (-146.3193, 3.1864) -> (-146.85, 3.2774)
  line L544 (-148.996, 7.5338) -> (-148.7536, 8.0147)
  line L545 (-148.7536, 8.0147) -> (-148.4334, 8.4476)
  line L546 (-149.0858, 5.4203) -> (-149.1993, 5.9467)
  line L547 (-148.2469, 4.0578) -> (-148.6027, 4.462)
  line L548 (-146.85, 3.2774) -> (-147.3578, 3.4568)
  line L549 (-147.3578, 3.4568) -> (-147.8279, 3.7195)
  line L550 (-147.8279, 3.7195) -> (-148.2469, 4.0578)
  line L551 (-148.6027, 4.462) -> (-148.885, 4.9206)
  line L552 (-148.885, 4.9206) -> (-149.0858, 5.4203)
  line L553 (-149.2214, 6.4847) -> (-149.1537, 7.0189)
  line L554 (-149.1993, 5.9467) -> (-149.2214, 6.4847)
  line L555 (-173.2279, 86.2695) -> (-173.6469, 86.6078)
  line L556 (-170.65, 85.8274) -> (-171.1807, 85.7364)
  line L557 (-168.3007, 88.4967) -> (-168.4142, 87.9703)
  line L558 (-171.45, 92.075) -> (-170.9134, 92.0293)
  line L559 (-169.6721, 86.2695) -> (-170.1422, 86.0069)
  line L560 (-171.1807, 85.7364) -> (-171.7193, 85.7364)
  line L561 (-174.1536, 90.5647) -> (-173.8334, 90.9969)
  line L562 (-173.6469, 86.6078) -> (-174.0027, 87.012)
  line L563 (-174.5993, 88.4967) -> (-174.6222, 89.0348)
  line L564 (-170.9134, 92.0293) -> (-170.3923, 91.8936)
  line L565 (-174.285, 87.4706) -> (-174.4858, 87.9703)
  line L566 (-169.9016, 91.6718) -> (-169.4554, 91.3703)
  line L567 (-174.6222, 89.0348) -> (-174.553, 89.5689)
  line L568 (-169.0666, 90.9976) -> (-168.7464, 90.5647)
  line L569 (-168.2779, 89.0348) -> (-168.3007, 88.4967)
  line L570 (-168.4142, 87.9703) -> (-168.615, 87.4706)
  line L571 (-171.9866, 92.0293) -> (-171.45, 92.075)
  line L572 (-168.7464, 90.5647) -> (-168.504, 90.0838)
  line L573 (-170.3923, 91.8936) -> (-169.9016, 91.6718)
  line L574 (-173.4446, 91.3703) -> (-172.9984, 91.6718)
  line L575 (-168.8973, 87.012) -> (-169.2531, 86.6078)
  line L576 (-173.8334, 90.9969) -> (-173.4446, 91.3703)
  line L577 (-174.4858, 87.9703) -> (-174.5993, 88.4967)
  line L578 (-174.396, 90.0838) -> (-174.1536, 90.5647)
  line L579 (-168.615, 87.4706) -> (-168.8973, 87.012)
  line L580 (-169.4554, 91.3703) -> (-169.0666, 90.9976)
  line L581 (-172.7578, 86.0069) -> (-173.2279, 86.2695)
  line L582 (-172.9984, 91.6718) -> (-172.5077, 91.8936)
  line L583 (-174.0027, 87.012) -> (-174.285, 87.4706)
  line L584 (-172.25, 85.8274) -> (-172.7578, 86.0069)
  line L585 (-169.2531, 86.6078) -> (-169.6721, 86.2695)
  line L586 (-168.504, 90.0838) -> (-168.3463, 89.5689)
  line L587 (-171.7193, 85.7364) -> (-172.25, 85.8274)
  line L588 (-174.553, 89.5689) -> (-174.396, 90.0838)
  line L589 (-172.5077, 91.8936) -> (-171.9866, 92.0293)
  line L590 (-170.1422, 86.0069) -> (-170.65, 85.8274)
  line L591 (-168.3463, 89.5689) -> (-168.2779, 89.0348)
  line L592 (-32.55, 168.3774) -> (-33.0578, 168.5569)
  line L593 (-32.8077, 174.4436) -> (-32.2866, 174.5793)
  line L594 (-32.2866, 174.5793) -> (-31.7496, 174.625)
  line L595 (-29.9721, 168.8195) -> (-30.4422, 168.5569)
  line L596 (-34.8993, 171.0467) -> (-34.9221, 171.5848)
  line L597 (-34.1334, 173.5476) -> (-33.7446, 173.9203)
  line L598 (-31.2134, 174.5793) -> (-30.6923, 174.4436)
  line L599 (-30.2016, 174.2218) -> (-29.7554, 173.9203)
  line L600 (-33.5279, 168.8195) -> (-33.9469, 169.1578)
  line L601 (-28.7142, 170.5203) -> (-28.915, 170.0206)
  line L602 (-33.0578, 168.5569) -> (-33.5279, 168.8195)
  line L603 (-29.1973, 169.5621) -> (-29.5531, 169.1578)
  line L604 (-29.0464, 173.1147) -> (-28.804, 172.6338)
  line L605 (-28.915, 170.0206) -> (-29.1973, 169.5621)
  line L606 (-34.3019, 169.5621) -> (-34.585, 170.0206)
  line L607 (-34.4536, 173.1147) -> (-34.1334, 173.5476)
  line L608 (-34.9221, 171.5848) -> (-34.8537, 172.1189)
  line L609 (-33.9469, 169.1578) -> (-34.3019, 169.5621)
  line L610 (-33.2984, 174.2218) -> (-32.8077, 174.4436)
  line L611 (-31.7496, 174.625) -> (-31.2134, 174.5793)
  line L612 (-34.7858, 170.5203) -> (-34.8993, 171.0467)
  line L613 (-30.6923, 174.4436) -> (-30.2016, 174.2218)
  line L614 (-29.5531, 169.1578) -> (-29.9721, 168.8195)
  line L615 (-29.3666, 173.5476) -> (-29.0464, 173.1147)
  line L616 (-28.804, 172.6338) -> (-28.6463, 172.1189)
  line L617 (-29.7554, 173.9203) -> (-29.3666, 173.5476)
  line L618 (-32.0193, 168.2864) -> (-32.55, 168.3774)
  line L619 (-30.4422, 168.5569) -> (-30.95, 168.3774)
  line L620 (-30.95, 168.3774) -> (-31.4807, 168.2864)
  line L621 (-31.4807, 168.2864) -> (-32.0193, 168.2864)
  line L622 (-34.585, 170.0206) -> (-34.7858, 170.5203)
  line L623 (-28.5779, 171.5848) -> (-28.6007, 171.0467)
  line L624 (-34.8537, 172.1189) -> (-34.696, 172.6338)
  line L625 (-28.6463, 172.1189) -> (-28.5779, 171.5848)
  line L626 (-34.696, 172.6338) -> (-34.4536, 173.1147)
  line L627 (-28.6007, 171.0467) -> (-28.7142, 170.5203)
  line L628 (-33.7446, 173.9203) -> (-33.2984, 174.2218)
  line L629 (-7.6578, 86.0069) -> (-8.1279, 86.2695)
  line L630 (-6.8866, 92.0293) -> (-6.35, 92.075)
  line L631 (-7.4077, 91.8936) -> (-6.8866, 92.0293)
  line L632 (-6.35, 92.075) -> (-5.8134, 92.0293)
  line L633 (-9.3858, 87.9703) -> (-9.4993, 88.4967)
  line L634 (-3.2463, 89.5682) -> (-3.1779, 89.0348)
  line L635 (-3.404, 90.0838) -> (-3.2463, 89.5682)
  line L636 (-4.3554, 91.3703) -> (-3.9666, 90.9976)
  line L637 (-3.9666, 90.9976) -> (-3.6464, 90.5647)
  line L638 (-5.8134, 92.0293) -> (-5.2923, 91.8936)
  line L639 (-4.8016, 91.6718) -> (-4.3554, 91.3703)
  line L640 (-5.2923, 91.8936) -> (-4.8016, 91.6718)
  line L641 (-3.6464, 90.5647) -> (-3.404, 90.0838)
  line L642 (-3.3142, 87.9703) -> (-3.515, 87.4706)
  line L643 (-3.1779, 89.0348) -> (-3.2007, 88.4967)
  line L644 (-3.2007, 88.4967) -> (-3.3142, 87.9703)
  line L645 (-3.515, 87.4706) -> (-3.7973, 87.012)
  line L646 (-3.7973, 87.012) -> (-4.1531, 86.6078)
  line L647 (-4.5721, 86.2695) -> (-5.0422, 86.0069)
  line L648 (-5.0422, 86.0069) -> (-5.55, 85.8274)
  line L649 (-4.1531, 86.6078) -> (-4.5721, 86.2695)
  line L650 (-5.55, 85.8274) -> (-6.0807, 85.7364)
  line L651 (-6.6193, 85.7364) -> (-7.15, 85.8274)
  line L652 (-6.0807, 85.7364) -> (-6.6193, 85.7364)
  line L653 (-7.15, 85.8274) -> (-7.6578, 86.0069)
  line L654 (-8.1279, 86.2695) -> (-8.5469, 86.6078)
  line L655 (-9.5221, 89.0348) -> (-9.4537, 89.5689)
  line L656 (-7.8984, 91.6718) -> (-7.4077, 91.8936)
  line L657 (-8.5469, 86.6078) -> (-8.9027, 87.012)
  line L658 (-8.9027, 87.012) -> (-9.185, 87.4706)
  line L659 (-9.0536, 90.5647) -> (-8.7334, 90.9969)
  line L660 (-9.4993, 88.4967) -> (-9.5221, 89.0348)
  line L661 (-9.4537, 89.5689) -> (-9.2961, 90.0838)
  line L662 (-8.7334, 90.9969) -> (-8.3446, 91.3703)
  line L663 (-8.3446, 91.3703) -> (-7.8984, 91.6718)
  line L664 (-9.185, 87.4706) -> (-9.3858, 87.9703)
  line L665 (-9.2961, 90.0838) -> (-9.0536, 90.5647)
  line L666 (-85.8642, 170.5203) -> (-86.065, 170.0206)
  line L667 (-85.7507, 171.0467) -> (-85.8642, 170.5203)
  line L668 (-86.7031, 169.1578) -> (-87.1221, 168.8195)
  line L669 (-85.954, 172.6338) -> (-85.7963, 172.1181)
  line L670 (-87.8423, 174.4436) -> (-87.3516, 174.2218)
  line L671 (-86.3473, 169.5621) -> (-86.7031, 169.1578)
  line L672 (-87.1221, 168.8195) -> (-87.5922, 168.5569)
  line L673 (-86.9054, 173.9203) -> (-86.5166, 173.5476)
  line L674 (-87.3516, 174.2218) -> (-86.9054, 173.9203)
  line L675 (-86.1964, 173.1147) -> (-85.954, 172.6338)
  line L676 (-88.3634, 174.5793) -> (-87.8423, 174.4436)
  line L677 (-85.7963, 172.1181) -> (-85.7279, 171.5848)
  line L678 (-86.065, 170.0206) -> (-86.3473, 169.5621)
  line L679 (-92.0493, 171.0467) -> (-92.0721, 171.5848)
  line L680 (-92.0721, 171.5848) -> (-92.0037, 172.1189)
  line L681 (-86.5166, 173.5476) -> (-86.1964, 173.1147)
  line L682 (-85.7279, 171.5848) -> (-85.7507, 171.0467)
  line L683 (-89.7, 168.3774) -> (-90.207, 168.5569)
  line L684 (-91.4527, 169.5621) -> (-91.735, 170.0206)
  line L685 (-90.6779, 168.8195) -> (-91.0969, 169.1578)
  line L686 (-89.1693, 168.2864) -> (-89.7, 168.3774)
  line L687 (-91.9358, 170.5203) -> (-92.0493, 171.0467)
  line L688 (-91.0969, 169.1578) -> (-91.4527, 169.5621)
  line L689 (-91.6036, 173.1147) -> (-91.2834, 173.5476)
  line L690 (-89.9577, 174.4436) -> (-89.4358, 174.5793)
  line L691 (-88.1, 168.3774) -> (-88.6307, 168.2864)
  line L692 (-87.5922, 168.5569) -> (-88.1, 168.3774)
  line L693 (-90.4484, 174.2218) -> (-89.9577, 174.4436)
  line L694 (-92.0037, 172.1189) -> (-91.846, 172.6338)
  line L695 (-90.8946, 173.9203) -> (-90.4484, 174.2218)
  line L696 (-90.207, 168.5569) -> (-90.6779, 168.8195)
  line L697 (-88.9, 174.625) -> (-88.3634, 174.5793)
  line L698 (-89.4358, 174.5793) -> (-88.9, 174.625)
  line L699 (-91.2834, 173.5476) -> (-90.8946, 173.9203)
  line L700 (-88.6307, 168.2864) -> (-89.1693, 168.2864)
  line L701 (-91.846, 172.6338) -> (-91.6036, 173.1147)
  line L702 (-91.735, 170.0206) -> (-91.9358, 170.5203)
  line L703 (-33.2984, 9.1218) -> (-32.8077, 9.3436)
  line L704 (-33.7446, 8.8203) -> (-33.2984, 9.1218)
  line L705 (-28.7142, 5.4203) -> (-28.915, 4.9206)
  line L706 (-32.2866, 9.4793) -> (-31.75, 9.525)
  line L707 (-31.2134, 9.4793) -> (-30.6923, 9.3436)
  line L708 (-32.55, 3.2774) -> (-33.057, 3.4568)
  line L709 (-29.0464, 8.0139) -> (-28.804, 7.5338)
  line L710 (-29.7554, 8.8203) -> (-29.3666, 8.4476)
  line L711 (-31.75, 9.525) -> (-31.2134, 9.4793)
  line L712 (-30.6923, 9.3436) -> (-30.2016, 9.1218)
  line L713 (-29.3666, 8.4476) -> (-29.0464, 8.0139)
  line L714 (-33.057, 3.4568) -> (-33.5272, 3.7195)
  line L715 (-30.2016, 9.1218) -> (-29.7554, 8.8203)
  line L716 (-33.9462, 4.0578) -> (-34.3027, 4.462)
  line L717 (-34.1334, 8.4469) -> (-33.7446, 8.8203)
  line L718 (-32.8077, 9.3436) -> (-32.2866, 9.4793)
  line L719 (-34.696, 7.5338) -> (-34.4536, 8.0147)
  line L720 (-28.6007, 5.9467) -> (-28.7142, 5.4203)
  line L721 (-30.95, 3.2774) -> (-31.4807, 3.1864)
  line L722 (-29.1973, 4.462) -> (-29.5531, 4.0578)
  line L723 (-34.7858, 5.4203) -> (-34.8993, 5.9467)
  line L724 (-34.8537, 7.0189) -> (-34.696, 7.5338)
  line L725 (-28.804, 7.5338) -> (-28.6463, 7.0189)
  line L726 (-34.4536, 8.0147) -> (-34.1334, 8.4469)
  line L727 (-32.0193, 3.1864) -> (-32.55, 3.2774)
  line L728 (-28.6463, 7.0189) -> (-28.5779, 6.4847)
  line L729 (-31.4807, 3.1864) -> (-32.0193, 3.1864)
  line L730 (-33.5272, 3.7195) -> (-33.9462, 4.0578)
  line L731 (-34.9221, 6.4847) -> (-34.8537, 7.0189)
  line L732 (-29.9721, 3.7195) -> (-30.4422, 3.4568)
  line L733 (-30.4422, 3.4568) -> (-30.95, 3.2774)
  line L734 (-28.5779, 6.4847) -> (-28.6007, 5.9467)
  line L735 (-34.3027, 4.462) -> (-34.585, 4.9206)
  line L736 (-34.585, 4.9206) -> (-34.7858, 5.4203)
  line L737 (-29.5531, 4.0578) -> (-29.9721, 3.7195)
  line L738 (-28.915, 4.9206) -> (-29.1973, 4.462)
  line L739 (-34.8993, 5.9467) -> (-34.9221, 6.4847)
  line L740 (-104.5689, 30.4322) -> (-104.6129, 30.8093)
  line L741 (-102.3838, 25.1347) -> (-102.7972, 25.1012)
  line L742 (-104.65, 25.9065) -> (-104.9078, 26.232)
  line L743 (-165.1, 165.0993) -> (-165.0911, 165.0993)
  line L744 (-104.14, 76.2) -> (-104.1387, 76.1999)
  line L745 (-104.3434, 25.6282) -> (-104.65, 25.9065)
  line L746 (-102.7972, 25.1012) -> (-103.2114, 25.1362)
  line L747 (-103.7337, 76.1686) -> (-103.3462, 76.0756)
  line L748 (-102.9787, 75.9231) -> (-102.6388, 75.7148)
  line L749 (-158.75, 165.0999) -> (-158.741, 165.0999)
  line L750 (-158.741, 165.0999) -> (-158.741, 76.2)
  line L751 (-105.2684, 28.2195) -> (-105.1403, 28.6153)
  line L752 (-104.6129, 30.8093) -> (-104.7125, 31.1756)
  line L753 (-165.0993, 44.45) -> (-165.1, 81.4578)
  line L754 (-101.5918, 73.6599) -> (-101.5918, 25.3999)
  line L755 (-102.3357, 75.4559) -> (-102.0761, 75.1529)
  line L756 (-165.1, 81.4578) -> (-165.0993, 101.1047)
  line L757 (-105.2494, 26.986) -> (-105.3233, 27.3945)
  line L758 (-165.0993, 101.1047) -> (-165.1, 161.4297)
  line L759 (-165.0911, 165.0999) -> (-161.9553, 165.0999)
  line L760 (-104.9078, 26.232) -> (-105.1091, 26.595)
  line L761 (-102.0761, 75.1529) -> (-101.8679, 74.813)
  line L762 (-103.3462, 76.0756) -> (-102.9787, 75.9231)
  line L763 (-101.981, 25.2352) -> (-102.3838, 25.1347)
  line L764 (-105.3233, 27.3945) -> (-105.3234, 27.4001)
  line L765 (-165.1, 161.4297) -> (-165.1, 165.0993)
  line L766 (-104.1387, 76.1999) -> (-104.1318, 76.1999)
  line L767 (-105.329, 27.8096) -> (-105.2684, 28.2195)
  line L768 (-161.4297, 165.1) -> (-158.75, 165.1)
  line L769 (-161.9553, 165.0999) -> (-161.4297, 165.1)
  line L770 (-105.1091, 26.595) -> (-105.2494, 26.986)
  line L771 (-111.76, 44.45) -> (-165.0993, 44.45)
  line L772 (-104.5817, 30.0528) -> (-104.5689, 30.4322)
  line L773 (-103.6132, 25.2367) -> (-103.9939, 25.4022)
  line L774 (-105.3234, 27.4001) -> (-105.329, 27.8096)
  line L775 (-101.7154, 74.4448) -> (-101.6223, 74.0572)
  line L776 (-101.6223, 74.0572) -> (-101.5918, 73.6599)
  line L777 (-104.8656, 31.523) -> (-111.76, 44.45)
  line L778 (-104.7125, 31.1756) -> (-104.8656, 31.523)
  line L779 (-101.8679, 74.813) -> (-101.7154, 74.4448)
  line L780 (-104.1318, 76.1999) -> (-103.7337, 76.1686)
  line L781 (-165.0911, 165.0993) -> (-165.0911, 165.0999)
  line L782 (-102.6388, 75.7148) -> (-102.3357, 75.4559)
  line L783 (-158.741, 76.2) -> (-104.14, 76.2)
  line L784 (-103.9939, 25.4022) -> (-104.3434, 25.6282)
  line L785 (-101.6459, 25.3801) -> (-101.981, 25.2352)
  line L786 (-101.5918, 25.3999) -> (-101.6459, 25.3801)
  line L787 (-103.2114, 25.1362) -> (-103.6132, 25.2367)
  line L788 (-104.7749, 29.3207) -> (-104.6509, 29.6795)
  line L789 (-104.951, 28.9844) -> (-104.7749, 29.3207)
  line L790 (-104.6509, 29.6795) -> (-104.5817, 30.0528)
  line L791 (-158.75, 165.1) -> (-158.75, 165.0999)
  line L792 (-105.1403, 28.6153) -> (-104.951, 28.9844)
  line L793 (-101.8724, 102.9831) -> (-102.0807, 102.6432)
  line L794 (-101.5956, 104.1362) -> (-101.6268, 103.7381)
  line L795 (-102.3395, 102.3402) -> (-102.6426, 102.0806)
  line L796 (-102.6426, 102.0806) -> (-102.9824, 101.8723)
  line L797 (-102.9824, 101.8723) -> (-103.3507, 101.7198)
  line L798 (-102.0807, 102.6432) -> (-102.3395, 102.3402)
  line L799 (-101.6268, 103.7381) -> (-101.7199, 103.3506)
  line L800 (-12.6956, 158.7455) -> (-101.5956, 158.7455)
  line L801 (-148.9798, 104.9436) -> (-148.6224, 104.7324)
  line L802 (-149.7732, 105.1787) -> (-149.3668, 105.0937)
  line L803 (-152.6148, 102.3942) -> (-152.6242, 102.8085)
  line L804 (-151.3719, 104.85) -> (-150.9985, 105.0299)
  line L805 (-147.1992, 104.2668) -> (-146.8202, 104.2887)
  line L806 (-130.3457, 165.0955) -> (-12.6956, 165.0955)
  line L807 (-152.009, 104.321) -> (-151.7125, 104.6116)
  line L808 (-152.566, 103.2195) -> (-152.4415, 103.6155)
  line L809 (-152.4415, 103.6155) -> (-152.378, 103.741)
  line L810 (-151.5123, 104.752) -> (-151.3719, 104.85)
  line L811 (-130.3457, 161.4252) -> (-130.3457, 165.0955)
  line L812 (-104.1356, 101.5962) -> (-152.3956, 101.5962)
  line L813 (-146.4487, 104.3669) -> (-146.0931, 104.4995)
  line L814 (-148.6224, 104.7324) -> (-148.2968, 104.537)
  line L815 (-101.5956, 158.7455) -> (-101.5956, 104.1362)
  line L816 (-12.6956, 165.0955) -> (-12.6956, 161.4252)
  line L817 (-150.1879, 105.1965) -> (-149.7732, 105.1787)
  line L818 (-12.6956, 161.4244) -> (-12.6956, 158.7455)
  line L819 (-150.9985, 105.0299) -> (-150.6, 105.1464)
  line L820 (-151.7125, 104.6116) -> (-151.5123, 104.752)
  line L821 (-146.0931, 104.4995) -> (-130.345, 111.7555)
  line L822 (-148.2968, 104.537) -> (-147.9459, 104.3923)
  line L823 (-103.7382, 101.6267) -> (-104.1356, 101.5962)
  line L824 (-103.3507, 101.7198) -> (-103.7382, 101.6267)
  line L825 (-101.7199, 103.3506) -> (-101.8724, 102.9831)
  line L826 (-150.6, 105.1464) -> (-150.1879, 105.1965)
  line L827 (-147.5773, 104.3016) -> (-147.1992, 104.2668)
  line L828 (-146.8202, 104.2887) -> (-146.4487, 104.3669)
  line L829 (-152.6242, 102.8085) -> (-152.566, 103.2195)
  line L830 (-130.345, 111.7555) -> (-130.3457, 161.4252)
  line L831 (-152.3956, 101.5962) -> (-152.5379, 101.9862)
  line L832 (-147.9459, 104.3923) -> (-147.5773, 104.3016)
  line L833 (-149.3668, 105.0937) -> (-148.9798, 104.9436)
  line L834 (-152.2534, 103.986) -> (-152.009, 104.321)
  line L835 (-152.5379, 101.9862) -> (-152.6148, 102.3942)
  line L836 (-12.6956, 161.4252) -> (-12.6956, 161.4244)
  line L837 (-152.378, 103.741) -> (-152.2534, 103.986)
  line L838 (-165.0911, 165.0999) -> (-12.7, 165.0999)
  line L839 (-12.7, 165.0999) -> (-12.7, 12.7)
  line L840 (-12.7, 12.7) -> (-165.0911, 12.7)
  line L841 (-165.0911, 12.7) -> (-165.0911, 165.0999)
  line L842 (-102.1279, 102.056) -> (-75.8393, 102.056)
  line L843 (-75.8393, 102.056) -> (-75.8393, 75.8432)
  line L844 (-75.8393, 75.8432) -> (-102.1279, 75.8432)
  line L845 (-102.1279, 75.8432) -> (-102.1279, 102.056)
  constraint horizontal L838
  constraint vertical L839
  constraint horizontal L840
  constraint vertical L841
  constraint horizontal L842
  constraint vertical L843
  constraint horizontal L844
  constraint vertical L845
extrude "Extrude1" add sketch "sdfjkvcsd" against normal blind 13 contours L0 L1 L2 L3 L4 L5 L6 L7 L8 L9 L10 L11 L12 | L14 L15 L16 L41 L42 L43 L44 L45 L46 L47 L48 L49 L50 L52 L53 L54 L55 L56 L57 L58 L59 L60 L61 L62 L63 L64 L65 L66 L67 L68 L69 L70 L71 L74 L75 L76 L77 L78 L79 L80 L81 L82 L85 L86 L87 L88 L89 L90 L91 L92 L93 L94 L95 L96 L97 L98 L99 L100 L101 L102 L103 L105 L107 L108 L109 L110 L111 L112 L113 L114 L115 L116 L117 L118 L119 L120 L121 L123 L124 L125 L126 L127 L128 L129 L130 L131 L133 L134 L135 L136 L138 L276 L277 L279 L329 L330 L332 L740 L741 L742 L745 L746 L747 L748 L750 L751 L752 L754 L755 L757 L760 L761 L762 L763 L764 L766 L767 L770 L771 L772 L773 L774 L775 L776 L777 L778 L779 L780 L782 L783 L784 L785 L786 L787 L788 L789 L790 L792 L793 L794 L795 L796 L797 L798 L799 L800 L801 L802 L803 L804 L805 L806 L807 L808 L809 L810 L811 L812 L813 L814 L815 L817 L819 L820 L821 L822 L823 L824 L825 L826 L827 L828 L829 L830 L831 L832 L833 L834 L835 L837 L838 L839 L840 L841 | L17 L23 L24 L26 L28 L30 L34 L39 L40 L251 L252 L255 L256 L264 L266 L271 L272 L274 L283 L284 L285 L286 L288 L295 L298 L299 L301 L305 L308 L310 L312 L315 L317 L318 L319 L320 L322 L325 L842 L843 L844 L845 makes body 1
extrude "Extrude6" add sketch "sdfjkvcsd" along normal blind 13 from surface at 10 separate body contours L0 L1 L2 L3 L4 L5 L6 L7 L8 L9 L10 L11 L12 | L14 L15 L16 L41 L42 L43 L44 L45 L46 L47 L48 L49 L50 L52 L53 L54 L55 L56 L57 L58 L59 L60 L61 L62 L63 L64 L65 L66 L67 L68 L69 L70 L71 L74 L75 L76 L77 L78 L79 L80 L81 L82 L85 L86 L87 L88 L89 L90 L91 L92 L93 L94 L95 L96 L97 L98 L99 L100 L101 L102 L103 L105 L107 L108 L109 L110 L111 L112 L113 L114 L115 L116 L117 L118 L119 L120 L121 L123 L124 L125 L126 L127 L128 L129 L130 L131 L133 L134 L135 L136 L138 L276 L277 L279 L329 L330 L332 L740 L741 L742 L745 L746 L747 L748 L750 L751 L752 L754 L755 L757 L760 L761 L762 L763 L764 L766 L767 L770 L771 L772 L773 L774 L775 L776 L777 L778 L779 L780 L782 L783 L784 L785 L786 L787 L788 L789 L790 L792 L793 L794 L795 L796 L797 L798 L799 L800 L801 L802 L803 L804 L805 L806 L807 L808 L809 L810 L811 L812 L813 L814 L815 L817 L819 L820 L821 L822 L823 L824 L825 L826 L827 L828 L829 L830 L831 L832 L833 L834 L835 L837 L838 L839 L840 L841 | L17 L23 L24 L26 L28 L30 L34 L39 L40 L251 L252 L255 L256 L264 L266 L271 L272 L274 L283 L284 L285 L286 L288 L295 L298 L299 L301 L305 L308 L310 L312 L315 L317 L318 L319 L320 L322 L325 L842 L843 L844 L845 makes body 2
extrude "Extrude7" add sketch "sdfjkvcsd" along normal blind 3.196 contours L17 L23 L24 L26 L28 L30 L34 L39 L40 L251 L252 L255 L256 L264 L266 L271 L272 L274 L283 L284 L285 L286 L288 L295 L298 L299 L301 L305 L308 L310 L312 L315 L317 L318 L319 L320 L322 L325 L842 L843 L844 L845 bodies 1